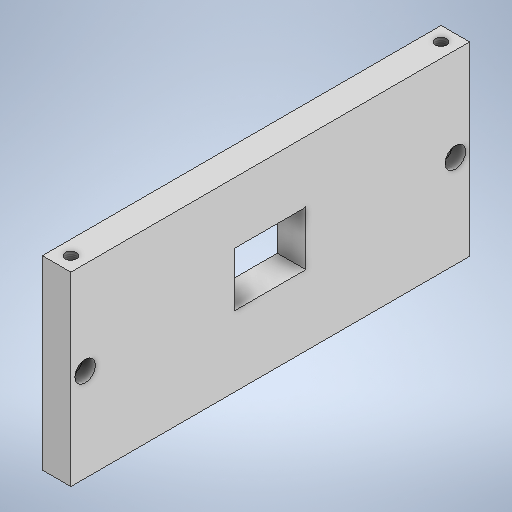
# Autodesk Inventor part: Rb PEEK - Largo
Saved by Autodesk Inventor 2025.1 (Build 291241000, 241)
## iProperties
Created: 2025-05-09
Part Number: Rb PEEK - Largo
Material: Generic
Document SubType Name: Modeling
Designer: E. Moreno
Density: 1 g/cm^3
Appearance: Default
Categories: <MemberInstance><Categories><Category DisplayName="" Mnemonic="CABLEANDHARNESS" InternalName="e4a7e005-5e42-4d16-b293-125e7f0d0512"><Category DisplayName="" Mnemonic="CONNECTORS" InternalName="6f634eba-a678-4820-a31d-2c2d5ee6728e"><CategoryParameter DisplayName="" Mnemonic="REFDES" InternalName="c3740e8c-60ab-4d5d-8584-52b73222f2f0"/><Category DisplayName="" Mnemonic="DISCRETEWIRE" InternalName="9a3407de-09b2-4cdb-8c40-9708d5144a28"/></Category></Category></Categories><FamilyTemplate><FamilyTemplateParameters></FamilyTemplateParameters></FamilyTemplate><CategoryParameterMap><ParamToTemplateMap><ParamToTemplate CategoryParameter="//CategoryParameter[@InternalName='c3740e8c-60ab-4d5d-8584-52b73222f2f0']" ConstantValue=""/></ParamToTemplateMap></CategoryParameterMap></MemberInstance>
Author: E. Moreno
Title: Rb PEEK - Largo
Autodesk Inventor part; units mm, degrees
ref_plane "YZ Plane" through (0, 0, 0) normal (1, 0, 0) x (0, 1, 0)
ref_plane "XZ Plane" through (0, 0, 0) normal (0, 1, 0) x (-1, 0, 0)
ref_plane "XY Plane" through (0, 0, 0) normal (0, 0, 1) x (1, 0, 0)
sketch "Sketch1" plane through (0, 0, 0) normal (1, 0, 0) x (0, 1, 0)
  line L0 (-32.6, 70) -> (32.6, 70)
  line L1 (32.6, 70) -> (32.6, -70)
  line L2 (32.6, -70) -> (-32.6, -70)
  line L3 (-32.6, -70) -> (-32.6, 70)
  line L4 (-32.6, 70) -> (32.6, -70) construction
  line L5 (32.6, 70) -> (-32.6, -70) construction
  point P0 (0, 0)
  dimension "d0" = 65.2
  dimension "d1" = 140
  constraints: 12 end point, 2 midpoint, 2 parallel, 1 horizontal, 1 perpendicular
  measures "d0" distance of L1.end L2.end
  measures "d1" distance of L0.end L1.end
extrude "Extrusion1" add sketch "Sketch1" along normal blind 10
sketch "Sketch2" plane through (0, 32.6, 70) normal (0, 1, 0) x (1, 0, 0)
  line L0 (0, 0) -> (10, 0) projected
  line L1 (0, 0) -> (5, 0)
  line L2 (5, 0) -> (5, 5)
  circle A0 centre (5, 5) radius 2
  line L3 (0, 70) -> (10, 70)
  line L4 (0, 140) -> (10, 140)
  line L5 (0, 140) -> (5, 140)
  line L6 (5, 140) -> (5, 135)
  circle A1 centre (5, 135) radius 2
  dimension "d4" = 5
  dimension "d5" = 5
  dimension "d6" = 4
  constraints: 12 end point, 5 symmetric about line, 2 centre point, 2 coincident, 1 horizontal, 1 midpoint, 1 perpendicular, 1 other
  measures "d4" distance of L0.start L1.end
  measures "d5" distance of L1.end L2.end
  measures "d6" diameter of A0
extrude "Extrusion2" cut sketch "Sketch2" against normal blind 25
thread "Thread1" size "M4x0.7" class "6H" standard "ANSI Metric M Profile" full length
thread "Thread2" size "M4x0.7" class "6H" standard "ANSI Metric M Profile" full length
sketch "Sketch3" plane through (0, -32.6, -70) normal (0, -1, 0) x (1, 0, 0)
  line L0 (0, 70) -> (9.9068, 70)
  line L1 (10, 0) -> (10, 140) projected
  line L2 (10, 140) -> (5, 140)
  line L3 (0, 140) -> (10, 140) projected
  line L4 (5, 140) -> (5, 135)
  circle A0 centre (5, 135) radius 2
  line L5 (10, 0) -> (5, 0)
  line L6 (0, 0) -> (10, 0)
  line L7 (5, 0) -> (5, 5)
  circle A1 centre (5, 5) radius 2
  dimension "d13" = 5
  dimension "d14" = 5
  dimension "d15" = 4
  constraints: 12 end point, 4 symmetric about line, 2 centre point, 2 coincident, 1 horizontal, 1 midpoint, 1 perpendicular, 1 other
  measures "d13" distance of L1.end L2.end
  measures "d14" distance of L2.end L4.end
  measures "d15" diameter of A0
extrude "Extrusion3" cut sketch "Sketch3" against normal blind 25
sketch "Sketch4" plane through (10, 0, 0) normal (1, 0, 0) x (0, 0, -1)
  line L0 (-70, 32.6) -> (-70, -32.6) projected
  line L1 (-70, 0) -> (-65, 0)
  circle A0 centre (-65, 0) radius 2
  line L2 (-70, -32.6) -> (70, -32.6) projected
  line L3 (0, -32.6) -> (0, 32.6)
  line L4 (70, 32.6) -> (-70, 32.6) projected
  line L5 (70, 0) -> (65, 0)
  circle A1 centre (65, 0) radius 2
  point P0 (0, 0)
  dimension "d18" = 5
  dimension "d19" = 4
  constraints: 6 end point, 3 midpoint, 3 symmetric about line, 2 centre point, 2 coincident, 1 horizontal, 1 other
  measures "d18" distance of L1.start L1.end
  measures "d19" diameter of A0
extrude "Extrusion4" cut sketch "Sketch4" against normal blind 10 contours A0 | A1
sketch "Sketch5" plane through (10, 0, 0) normal (1, 0, 0) x (0, 0, -1)
  circle A0 centre (-65, 0) radius 3.61
  circle A1 centre (-65, 0) radius 2 projected
  line L0 (0, 33.0095) -> (0, -32.6)
  line L1 (-70, -32.6) -> (70, -32.6) projected
  circle A2 centre (65, 0) radius 3.61
  circle A3 centre (65, 0) radius 2
  point P0 (0, 0)
  dimension "d22" = 7.22
  constraints: 3 centre point, 2 end point, 2 symmetric about line, 1 concentric, 1 midpoint, 2 other
  measures "d22" diameter of A0
extrude "Extrusion5" cut sketch "Sketch5" against normal blind 4.5
thread "Thread3" size "M4x0.7" class "6H" standard "ANSI Metric M Profile" full length
thread "Thread4" size "M4x0.7" class "6H" standard "ANSI Metric M Profile" full length
sketch "Sketch6" plane through (10, 0, 0) normal (1, 0, 0) x (0, 0, -1)
  line L0 (-70, -32.6) -> (70, -32.6) projected
  line L1 (0, -32.6) -> (0, 1.6)
  line L2 (-12.5, -7.9) -> (12.5, -7.9)
  line L3 (12.5, -7.9) -> (12.5, 11.1)
  line L4 (12.5, 11.1) -> (-12.5, 11.1)
  line L5 (-12.5, 11.1) -> (-12.5, -7.9)
  line L6 (-12.5, -7.9) -> (12.5, 11.1) construction
  line L7 (12.5, -7.9) -> (-12.5, 11.1) construction
  point P0 (0, 0)
  dimension "d29" = 34.2
  dimension "d30" = 25
  dimension "d31" = 19
  constraints: 14 end point, 3 midpoint, 2 parallel, 1 horizontal, 1 perpendicular, 1 vertical
  measures "d29" distance of L1.start L1.end
  measures "d30" distance of L4.end L3.end
  measures "d31" distance of L3.end L2.end
extrude "Extrusion6" cut sketch "Sketch6" against normal blind 10
sketch "Sketch10" plane through (10, 0, 0) normal (1, 0, 0) x (0, 0, -1)
  circle A0 centre (-27.5, 25.1) radius 2.5 projected
sketch "Sketch11" plane through (0, 0, 0) normal (-1, 0, 0) x (0, 0, 1)
  circle A0 centre (27.5, 25.1) radius 2.5 projected
body "Solid1"
